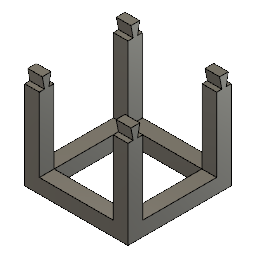
impossible cube (~recovered) (Autodesk Fusion 360 design; units mm, degrees)
Autodesk Fusion 360 part; units mm, degrees
sketch "Sketch1" plane through (0, 0, 0) normal (0, 1, 0) x (1, 0, 0)
  line L0 (5.1128, -4.9272) -> (94.0128, -4.9272)
  line L1 (94.0128, -4.9272) -> (94.0128, -93.8272)
  line L2 (94.0128, -93.8272) -> (5.1128, -93.8272)
  line L3 (5.1128, -93.8272) -> (5.1128, -4.9272)
  line L4 (17.8128, -17.6272) -> (81.3128, -17.6272)
  line L5 (81.3128, -17.6272) -> (81.3128, -81.1272)
  line L6 (81.3128, -81.1272) -> (17.8128, -81.1272)
  line L7 (17.8128, -81.1272) -> (17.8128, -17.6272)
  dimension "d1" = 88.9
  dimension "d2" = 88.9
  dimension "d3" = 12.7
  dimension "d4" = 12.7
  dimension "d5" = 12.7
  dimension "d6" = 12.7
  constraint horizontal L0
  constraint vertical L1
  constraint horizontal L2
  constraint vertical L3
  constraint horizontal L4
  constraint vertical L5
  constraint horizontal L6
  constraint vertical L7
  measures "d1" distance of L0.start L0.end
  measures "d2" distance of L0.start L2.end
  measures "d3" distance of L1 L5
  measures "d4" distance of L3 L7
  measures "d5" distance of L2 L6
  measures "d6" distance of L0 L4
extrude "Extrude1" add sketch "Sketch1" along normal blind 88.9
sketch "Sketch2" plane through (0, 0, 93.8272) normal (0, 0, 1) x (1, 0, 0)
  line L0 (5.1128, 0) -> (94.0128, 0)
  line L1 (94.0128, 0) -> (94.0128, 88.9)
  line L2 (94.0128, 88.9) -> (5.1128, 88.9)
  line L3 (5.1128, 88.9) -> (5.1128, 0)
  line L4 (17.8128, 76.2) -> (81.3128, 76.2)
  line L5 (81.3128, 76.2) -> (81.3128, 12.7)
  line L6 (81.3128, 12.7) -> (17.8128, 12.7)
  line L7 (17.8128, 12.7) -> (17.8128, 76.2)
  dimension "d9" = 12.7
  dimension "d10" = 12.7
  dimension "d11" = 12.7
  dimension "d12" = 12.7
  constraint horizontal L4
  constraint vertical L5
  constraint horizontal L6
  constraint vertical L7
  measures "d9" distance of L2 L4
  measures "d10" distance of L1 L5
  measures "d11" distance of L0 L6
  measures "d12" distance of L3 L7
extrude "Extrude2" cut sketch "Sketch2" against normal blind 88.9 contours L4 L5 L6 L7
sketch "Sketch3" plane through (5.1128, 0, 0) normal (-1, 0, 0) x (0, 0, 1)
  line L0 (4.9272, 0) -> (93.8272, 0)
  line L1 (93.8272, 0) -> (93.8272, 88.9)
  line L2 (93.8272, 88.9) -> (4.9272, 88.9)
  line L3 (4.9272, 88.9) -> (4.9272, 0)
  line L4 (17.6272, 76.2) -> (81.1272, 76.2)
  line L5 (81.1272, 76.2) -> (81.1272, 12.7)
  line L6 (81.1272, 12.7) -> (17.6272, 12.7)
  line L7 (17.6272, 12.7) -> (17.6272, 76.2)
  dimension "d15" = 12.7
  dimension "d16" = 12.7
  dimension "d17" = 12.7
  dimension "d18" = 12.7
  constraint horizontal L4
  constraint vertical L5
  constraint horizontal L6
  constraint vertical L7
  measures "d15" distance of L2 L4
  measures "d16" distance of L1 L5
  measures "d17" distance of L0 L6
  measures "d18" distance of L3 L7
extrude "Extrude3" cut sketch "Sketch3" against normal blind 88.9 contours L4 L5 L6 L7
sketch "Sketch4" plane through (5.1128, 0, 0) normal (-1, 0, 0) x (0, 0, 1)
  line L0 (81.1272, 76.2) -> (81.1272, 12.7)
  line L1 (81.1272, 12.7) -> (17.6272, 12.7)
  line L2 (17.6272, 12.7) -> (17.6272, 76.2)
  line L3 (17.6272, 76.2) -> (81.1272, 76.2)
  line L4 (4.9272, 0) -> (93.8272, 0)
  line L5 (93.8272, 0) -> (93.8272, 88.9)
  line L6 (93.8272, 88.9) -> (4.9272, 88.9)
  line L7 (4.9272, 88.9) -> (4.9272, 0)
  line L8 (17.6272, 76.2) -> (81.1272, 76.2)
  line L9 (81.1272, 88.9) -> (17.6272, 88.9)
  line L10 (17.6272, 76.2) -> (4.9272, 76.2) construction
  line L11 (11.2772, 76.2) -> (11.2772, 88.9) construction
  line L12 (17.6272, 76.2) -> (13.1822, 76.2)
  line L13 (4.9272, 76.2) -> (9.3722, 76.2)
  line L14 (17.6272, 88.9) -> (15.0872, 88.9) construction
  line L15 (4.9272, 88.9) -> (7.4672, 88.9)
  line L16 (7.4672, 88.9) -> (7.4672, 86.36) construction
  line L17 (15.0872, 88.9) -> (15.0872, 86.36) construction
  line L18 (9.3722, 76.2) -> (7.4672, 86.36)
  line L19 (7.4672, 86.36) -> (15.0872, 86.36)
  line L20 (13.1822, 76.2) -> (15.0872, 86.36)
  line L21 (81.1272, 76.2) -> (93.8272, 76.2) construction
  line L22 (87.4772, 76.2) -> (87.4772, 88.9) construction
  line L23 (81.1272, 76.2) -> (85.5722, 76.2)
  line L24 (93.8272, 76.2) -> (89.3822, 76.2)
  line L25 (81.1272, 88.9) -> (83.6672, 88.9) construction
  line L26 (93.8272, 88.9) -> (91.2872, 88.9) construction
  line L27 (91.2872, 88.9) -> (91.2872, 86.36) construction
  line L28 (83.6672, 88.9) -> (83.6672, 86.36) construction
  line L29 (85.5722, 76.2) -> (83.6672, 86.36)
  line L30 (91.2872, 86.36) -> (89.3822, 76.2)
  line L31 (91.2872, 86.36) -> (83.6672, 86.36)
  dimension "d21" = 4.445
  dimension "d22" = 4.445
  dimension "d23" = 2.54
  dimension "d24" = 2.54
  dimension "d25" = 2.54
  dimension "d26" = 2.54
  dimension "d27" = 4.445
  dimension "d28" = 4.445
  dimension "d30" = 2.54
  dimension "d31" = 2.54
  dimension "d32" = 2.54
  constraint horizontal L8
  constraint horizontal L9
  constraint coincident L2.end L3.start
  constraint coincident L7 L10.end
  constraint perpendicular L7 L10
  constraint midpoint L10 L11.start
  constraint coincident L6 L11.end
  constraint perpendicular L6 L11
  constraint perpendicular L7 L13
  constraint coincident L6.end L7.start
  constraint perpendicular L7 L15
  constraint perpendicular L6 L16
  constraint perpendicular L14 L17
  constraint coincident L5 L21.end
  constraint perpendicular L5 L21
  constraint midpoint L21 L22.start
  constraint coincident L6 L22.end
  constraint perpendicular L6 L22
  constraint perpendicular L5 L24
  constraint coincident L5.end L6.start
  constraint perpendicular L5 L26
  constraint perpendicular L6 L27
  constraint perpendicular L25 L28
  measures "d21" distance of L2.end L12.end
  measures "d22" distance of L10.end L13.end
  measures "d23" distance of L9.end L14.end
  measures "d24" distance of L6.end L15.end
  measures "d25" distance of L15.end L16.end
  measures "d26" distance of L14.end L17.end
  measures "d27" distance of L0.start L23.end
  measures "d28" distance of L21.end L24.end
  measures "d30" distance of L5.end L26.end
  measures "d31" distance of L26.end L27.end
  measures "d32" distance of L25.end L28.end
sketch "Sketch5" plane through (0, 0, 4.9272) normal (0, 0, -1) x (-1, 0, 0)
  line L0 (-81.3128, 12.7) -> (-81.3128, 76.2)
  line L1 (-81.3128, 76.2) -> (-17.8128, 76.2)
  line L2 (-17.8128, 76.2) -> (-17.8128, 12.7)
  line L3 (-17.8128, 12.7) -> (-81.3128, 12.7)
  line L4 (-94.0128, 0) -> (-5.1128, 0)
  line L5 (-5.1128, 0) -> (-5.1128, 88.9)
  line L6 (-5.1128, 88.9) -> (-94.0128, 88.9)
  line L7 (-94.0128, 88.9) -> (-94.0128, 0)
  line L8 (-81.3128, 76.2) -> (-17.8128, 76.2)
  line L9 (-17.8128, 76.2) -> (-17.8128, 88.9)
  line L10 (-17.8128, 88.9) -> (-81.3128, 88.9)
  line L11 (-81.3128, 88.9) -> (-81.3128, 76.2)
  constraint horizontal L8
  constraint vertical L9
  constraint horizontal L10
  constraint vertical L11
  constraint coincident L6 L9.end
  constraint coincident L0.end L1.start
extrude "Extrude4" cut sketch "Sketch5" against normal blind 88.9 contours L1 L6 L8 L9 L10 L11
extrude "Extrude5" cut sketch "Sketch4" against normal blind 88.9 contours L3 L5 L6 L7 L8 L9 L12 L13 L15 L18 L19 L20 L23 L24 L29 L30 L31
